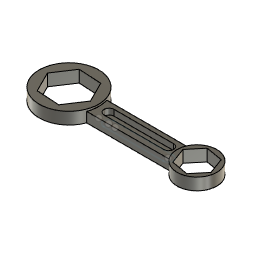
excersise 2 v1 (Autodesk Fusion 360 design; units mm, degrees)
Autodesk Fusion 360 part; units mm, degrees
sketch "Sketch1" plane through (0, 0, 0) normal (0, 0, 1) x (1, 0, 0) in component "ex2"
  circle A0 centre (0, 0) radius 30
  circle A1 centre (129, 0) radius 20
  line L0 (12.7246, 19.2722) -> (-10.328, 20.6559)
  line L1 (-10.328, 20.6559) -> (-23.0525, 1.3837)
  line L2 (-23.0525, 1.3837) -> (-12.7246, -19.2722)
  line L3 (-12.7246, -19.2722) -> (10.328, -20.6559)
  line L4 (10.328, -20.6559) -> (23.0525, -1.3837)
  line L5 (23.0525, -1.3837) -> (12.7246, 19.2722)
  line L6 (146.0675, -2.9498) -> (140.0883, 13.306)
  line L7 (140.0883, 13.306) -> (123.0208, 16.2558)
  line L8 (123.0208, 16.2558) -> (111.9325, 2.9498)
  line L9 (111.9325, 2.9498) -> (117.9117, -13.306)
  line L10 (117.9117, -13.306) -> (134.9792, -16.2558)
  line L11 (134.9792, -16.2558) -> (146.0675, -2.9498)
  line L12 (28.4216, 9.6028) -> (111.4561, 9.6028)
  line L13 (28.1407, -10.3972) -> (111.915, -10.3972)
  line L14 (70.2554, 9.6028) -> (70.2554, -10.3972) construction
  line L15 (40.1843, 5.2583) -> (100.1843, 5.2583)
  line L16 (100.1843, -4.7417) -> (40.1843, -4.7417)
  arc A2 (40.1843, 5.2583) -> (40.1843, -4.7417) centre (40.1843, 0.2583) ccw
  arc A3 (100.1843, -4.7417) -> (100.1843, 5.2583) centre (100.1843, 0.2583) ccw
  point P0 (129, 0)
  dimension "d1" = 60
  dimension "d2" = 40
  dimension "d3" = 129
  dimension "d4" = 20
  dimension "d5" = 15
  dimension "d6" = 20
  dimension "d9" = 60
  dimension "d10" = 10
  constraint coincident A0.centre origin
  constraint coincident P0 A1.centre
  constraint horizontal L12
  constraint horizontal L13
  constraint coincident A0 L13.start
  constraint coincident A1 L13.end
  constraint coincident A1 L12.end
  constraint coincident A0 L12.start
  constraint coincident L12 L14.start
  constraint perpendicular L12 L14
  constraint coincident L13 L14.end
  constraint horizontal L15
  constraint horizontal L16
  constraint tangent L16 A2
  constraint tangent L16 A3
  measures "d1" diameter of A0
  measures "d2" diameter of A1
  measures "d3" distance of A0.centre P0
  measures "d4" distance of A0.centre L5
  measures "d5" distance of P0 L11
  measures "d6" distance of L12 L13
  measures "d9" distance of L15.start L15.end
  measures "d10" distance of L15.start L16.end
extrude "Extrude1" add sketch "Sketch1" along normal blind 10 contours A0 A1 L12 L13 in component "ex2"
sketch "Sketch1 (2)" plane through (0, 0, 0) normal (0, 0, 1) x (1, 0, 0)
  line L0 (30, 0) -> (46.6152, 0) construction
  constraint horizontal L0
sketch "Sketch2" plane through (0, 0, 0) normal (0, 0, 1) x (1, 0, 0)
  line L0 (40, 5) -> (100, 5)
  line L1 (100, -5) -> (40, -5)
  arc A0 (40, 5) -> (40, -5) centre (40, 0) ccw
  arc A1 (100, -5) -> (100, 5) centre (100, 0) ccw
  dimension "d7" = 10
  dimension "d8" = 60
  constraint horizontal L0
  constraint horizontal L1
  constraint tangent L1 A0
  constraint tangent L1 A1
  measures "d7" distance of L0.start L1.end
  measures "d8" distance of L0.start L0.end
sketch "Sketch2 (2)" plane through (0, 0, 0) normal (0, 0, 1) x (1, 0, 0) in component "ex2"
extrude "Extrude2" add sketch "Sketch1" along normal blind 12 contours A0 | A1 in component "ex2"
extrude "Extrude3" add sketch "Sketch1" along normal blind 4 contours L15 L16 A2 A3 in component "ex2"
component "ex2" placed x (1, 0, 0) y (0, 1, 0) z (0, 0, 1) at (0, 0, 0)
